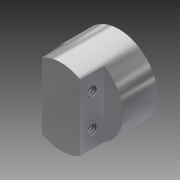
# Autodesk Inventor part: Pneumatic Connector - Side Side
Saved by Autodesk Inventor 2013 (Build 170138000, 138)
## iProperties
Created: 2013-06-08
Part Number: Pneumatic Connector - Side Side
Material: Generic
Document SubType Name: Modeling
Designer: mvarma
Density: 1 g/cm^3
Author: mvarma
Autodesk Inventor part; units mm, degrees
ref_plane "YZ Plane" through (0, 0, 0) normal (1, 0, 0) x (0, 1, 0)
ref_plane "XZ Plane" through (0, 0, 0) normal (0, 1, 0) x (-1, 0, 0)
ref_plane "XY Plane" through (0, 0, 0) normal (0, 0, 1) x (1, 0, 0)
sketch "Sketch1" plane through (0, 0, 0) normal (0, 0, 1) x (1, 0, 0)
  circle A0 centre (0, 0) radius 7.9375
  circle A1 centre (0, 0) radius 3.175
  circle A2 centre (0, 0) radius 12.7
  circle A3 centre (0, 0) radius 10.0965 construction
  line L0 (0, 0) -> (0, 10.0965) construction
  line L1 (0, 0) -> (0, -10.0965) construction
  circle A4 centre (0, 0) radius 6.35
  dimension "d0" = 15.875
  dimension "d1" = 6.35
  dimension "d2" = 25.4
  dimension "d4" = 2.159
  dimension "d5" = 12.7
  constraints: 7 coincident, 5 centre point, 4 end point, 2 point on circle, 1 collinear, 1 vertical
  measures "d0" diameter of A0
  measures "d1" diameter of A1
  measures "d2" diameter of A2
  measures "d4" radial gap between concentric circles of A0 A3
  measures "d5" diameter of A4
extrude "Extrusion1" add sketch "Sketch1" along normal blind 4.9784 contours A2
sketch "Sketch2" plane through (0, 0, 4.9784) normal (0, 0, 1) x (1, 0, 0)
  circle A0 centre (0, 0) radius 12.7 projected
  circle A1 centre (0, 0) radius 6.35 projected
extrude "Extrusion2" add sketch "Sketch2" along normal blind 3.175
sketch "Sketch3" plane through (0, 0, 8.1534) normal (0, 0, 1) x (1, 0, 0)
  circle A0 centre (0, 0) radius 12.7 projected
extrude "Extrusion3" add sketch "Sketch3" along normal blind 3.175
sketch "Sketch4" plane through (0, 0, 11.3284) normal (0, 0, 1) x (1, 0, 0)
  circle A0 centre (0, 0) radius 12.7 projected
  line L0 (-6.35, 10.9985) -> (-6.35, -10.9985)
  line L1 (6.35, 10.9985) -> (6.35, -10.9985)
  line L2 (0, 12.7) -> (0, -12.7) construction
  dimension "d12" = 6.35
  constraints: 6 end point, 6 point on circle, 2 parallel, 1 midpoint, 1 vertical, 1 other
  measures "d12" distance between parallel lines of L0 L2
extrude "Extrusion4" add sketch "Sketch4" along normal blind 7.9375 contours L1 A0 L0
sketch "Sketch5" plane through (-6.35, -10.9985, 11.3284) normal (-1, 0, 0) x (0, 0, 1)
  line L0 (0, 0) -> (0, 21.997) projected
  line L1 (0, 0) -> (7.9375, 0) projected
  line L2 (7.9375, 21.997) -> (7.9375, 0) projected
  line L3 (0, 21.997) -> (7.9375, 21.997) projected
  line L4 (7.9375, 10.9985) -> (0, 10.9985) construction
  line L5 (7.9375, 16.4978) -> (0, 16.4978) construction
  line L6 (0, 5.4993) -> (7.9375, 5.4993) construction
  line L7 (3.9688, 0) -> (3.9688, 21.997) construction
  point P0 (-11.3284, 10.9985)
  point P1 (3.9688, 16.4978)
  point P2 (3.9688, 5.4993)
  dimension "d15" = 5.4993
  dimension "d16" = 5.4993
  constraints: 8 end point, 6 midpoint, 6 point on line, 2 perpendicular, 1 other
  measures "d15" distance between parallel lines of L4 L5
  measures "d16" distance between parallel lines of L3 L5
hole "Hole1" at (-6.35, 5.4993, 15.2971) at (-6.35, -5.4993, 15.2971) direction (1, 0, 0) diameter 3.302 depth 25.4 tip angle 118 thread size "8-32 UNC" class "2B" standard "ANSI Unified Screw Threads"
hole "Hole2" at (0, 10.0965, 0) at (0, -10.0965, 0) direction (0, 0, 1) diameter 2.6416 depth 7.9375 tip angle 118 thread size "6-32 UNC" class "2B" standard "ANSI Unified Screw Threads"
equation "\"d15\" = d16"
body "Solid1"
